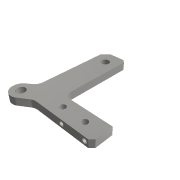
# Autodesk Inventor part: 100007
Saved by Autodesk Inventor 2020.1 (Build 241239000, 239)
## iProperties
MajorVersion: 11
MinorVersion: 1
Shininess: 64.0
Length Units: 11269
Angle Units: 11279
Time Units: 11290
Mass Units: 11283
Length Display Precision: 3
Angle Display Precision: 2
Compacted: True
Company: AUTODESK, INC.
Part Number: 100007
Document SubType Name: Modeling
Created: 2004-04-01
Designer: SCHNEIDER K.
Material: STEEL - MILD
Project: ADSK-000-000000
Description: LOCATER
Density: 7.86 g/cm^3
Appearance: Yellow
Density: 0.0
Volumn: 0.0
Area: 0.0
PropertySet Name: Model Information
Control State: 0
Master: False
Checked Out: False
Title: PLATE
Author: SCHNEIDER K.
Revision Number: -
Autodesk Inventor part; units mm, degrees
note: some values were not read from the file. Chosen so that the rebuilt part matches the saved one: edges of "面取り1".
ref_plane "YZ Plane" through (0, 0, 0) normal (1, 0, 0) x (0, 1, 0)
ref_plane "XZ Plane" through (0, 0, 0) normal (0, 1, 0) x (-1, 0, 0)
sketch "スケッチ2" plane through (0, 0, 0) normal (0, 0, 1) x (1, 0, 0)
  line L0 (-162.2425, 92.7575) -> (-162.2425, 62.7575)
  line L1 (-267.2425, 207.7575) -> (-237.2425, 207.7575)
  arc A0 (-290.563, 75.2382) -> (-273.922, 50.2767) centre (-282.2425, 62.7575) ccw
  line L2 (-277.2425, 84.1186) -> (-290.563, 75.2382)
  line L3 (-277.2425, 84.1186) -> (-277.2425, 197.7575)
  line L4 (-277.2425, 197.7575) -> (-267.2425, 207.7575)
  line L5 (-237.2425, 207.7575) -> (-237.2425, 92.7575)
  line L6 (-237.2425, 92.7575) -> (-162.2425, 92.7575)
  line L7 (-273.922, 50.2767) -> (-255.2008, 62.7575)
  line L8 (-255.2008, 62.7575) -> (-162.2425, 62.7575)
  line L9 (-282.2425, 62.7575) -> (-237.2425, 92.7575) construction
  point P0 (0, 0)
  point P1 (-277.2425, 207.7575)
  dimension "d18" = 120
  dimension "d21" = 15
  dimension "d22" = 10
  dimension "d23" = 10
  dimension "d116" = 5
  dimension "d154" = 15
  dimension "d155" = 145
  dimension "d175" = 30
  dimension "d181" = 90
  dimension "d182" = 40
  constraints: 20 end point, 5 parallel, 2 perpendicular, 2 point on circle, 2 point on line, 2 tangent, 1 centre point, 1 horizontal, 1 other
  measures "d18" distance from line of L0 L9.start
  measures "d21" radius of A0
  measures "d22" distance of L3.end point (-277.242, 207.757)
  measures "d23" distance of L1.start point (-277.242, 207.757)
  measures "d116" distance from line of L9.start L3
  measures "d154" distance edge to line of A0 L8
  measures "d155" distance from line of L1 L9.start
  measures "d175" distance between parallel lines of L6 L8
  measures "d181" angle of L8 L3
  measures "d182" distance between parallel lines of L5 L3
extrude "押し出し2" add sketch "スケッチ2" along normal blind 12
sketch "スケッチ3" plane through (0, 0, 12) normal (0, 0, 1) x (1, 0, 0)
  arc A0 (-290.563, 75.2382) -> (-282.2425, 47.7575) centre (-282.2425, 62.7575) ccw projected
  line L0 (-267.2425, 207.7575) -> (-237.2425, 207.7575) projected
  point P0 (-257.2425, 185.2575)
  dimension "d16" = 25
  dimension "d153" = 22.5
  constraints: 1 coincident
  measures "d16" horizontal distance of point (-282.242, 62.757) point (-257.242, 185.257)
  measures "d153" distance from line of L0 point (-257.242, 185.257)
hole "穴1" at (-257.2425, 185.2575, 12) at (-282.2425, 62.7575, 12) direction (0, 0, -1) diameter 14 end through all
sketch "スケッチ10" plane through (-237.2425, 92.7575, 0) normal (0, 1, 0) x (1, 0, 0)
  line L0 (75, 0) -> (75, -12)
  line L1 (0, -12) -> (75, -12)
  line L2 (75, 0) -> (0, 0) projected
  point P0 (65, -6)
  point P1 (30, -6)
  dimension "d119" = 35
  dimension "d156" = 10
  dimension "d157" = 6
  constraints: 4 end point, 1 horizontal alignment, 1 perpendicular
  measures "d119" distance of point (30, -6) point (65, -6)
  measures "d156" distance from line of L0 point (65, -6)
  measures "d157" distance from line of L1 point (30, -6)
hole "穴8" at (-172.2425, 92.7575, 6) at (-207.2425, 92.7575, 6) direction (0, -1, 0) diameter 6.6 end through all
chamfer "面取り1" distance 5 angle 45 1 edges at (-162.2425, 62.7575, 6)
fillet "フィレット1" radius 10 1 edges at (-237.2425, 92.7575, 6)
chamfer "面取り2" distance 5 angle 45 1 edges at (-237.2425, 207.7575, 6)
ref_plane "Work Plane2" through (-255.2008, 77.7575, 0) normal (0, -1, 0) x (1, 0, 0)
sketch "Sketch18" plane through (0, 0, 0) normal (0, 0, -1) x (-1, 0, 0)
  line L0 (162.2425, 67.7575) -> (162.2425, 92.7575) projected
  line L1 (324.2425, 77.7575) -> (135.2425, 77.7575) construction
  point P0 (187.2425, 77.7575)
  dimension "d165" = 25
  constraints: 1 point on line
  measures "d165" distance from line of L0 point (187.242, 77.757)
hole "Hole13" at (-187.2425, 77.7575, 0) direction (0, 0, 1) diameter 9 end through all
pattern_linear "Rectangular Pattern1" count 2 spacing 35 along (-1, 0, 0) of "Hole13"
fillet "Fillet2" radius 15 2 edges at (-255.2008, 62.7575, 6) (-277.2425, 84.1186, 6)
equation "\"d23\" = d22"
body "Solid1"
